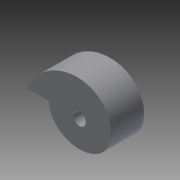
# Autodesk Inventor part: cam 2
Saved by Autodesk Inventor 2014 (Build 180170000, 170)
## iProperties
Created: 2014-05-19
Part Number: cam 2
Material: Generic
Document SubType Name: Modeling
Designer: jyesowitz
Density: 1 g/cm^3
Appearance: Default
Author: jyesowitz
Autodesk Inventor part; units mm, degrees
ref_plane "YZ Plane" through (0, 0, 0) normal (1, 0, 0) x (0, 1, 0)
ref_plane "XZ Plane" through (0, 0, 0) normal (0, 1, 0) x (-1, 0, 0)
ref_plane "XY Plane" through (0, 0, 0) normal (0, 0, 1) x (1, 0, 0)
sketch "Sketch1" plane through (0, 0, 0) normal (0, 0, 1) x (1, 0, 0)
  ellipse E0 centre (-0.0008, -0.0924) end of major axis (23.5196, -0.0924) minor radius 20.2596 (-23.521, 0) -> (22.8214, -4.992) ccw
  line L0 (22.8214, -4.992) -> (30.9811, 23.2074) construction
  line L1 (30.9811, 23.2074) -> (0.0058, 41.0577) construction
  line L2 (0.0058, 41.0577) -> (-30.9314, 23.2159) construction
  line L3 (-30.9314, 23.2159) -> (-40.386, 0) construction
  spline S0 degree 4 poles (22.8214, -4.992) (30.9811, 23.2074) (0.0058, 41.0577) (-30.9314, 23.2159) (-40.386, 0) knots 1 1 1 1 1 2 2 2 2 2
  line L4 (-40.386, 0) -> (-23.521, 0)
  circle A0 centre (-0.0008, -0.0924) radius 4.7625
  point P0 (0, 0)
  dimension "d60" = 23.5204
  dimension "d61" = 20.2596
  dimension "d18" = 40.386
  dimension "d19" = 16.865
  dimension "d29" = 41.0577
  dimension "d30" = 35.7133
  dimension "d31" = 25.0673
  dimension "d32" = 35.7507
  dimension "d33" = 29.3562
  dimension "d43" = 120.074
  dimension "d50" = 9.525
  dimension "d62" = 103.815
  dimension "d63" = 106.138
  constraints: 2 end point, 1 centre point, 1 coincident, 1 horizontal, 8 other
  measures "d18" distance of point (0, 0) L3.end
  measures "d19" distance of L3.end L4.end
  measures "d29" distance of L1.end point (0, 0)
  measures "d30" distance of L1.end L2.end
  measures "d31" distance of L2.end L3.end
  measures "d32" distance of L0.end L1.end
  measures "d33" distance of L0.start L0.end
  measures "d43" angle of L2 L1
  measures "d50" diameter of A0
  measures "d62" angle of L0 L1
  measures "d63" angle of L0 L4
extrude "Extrusion1" add sketch "Sketch1" against normal blind 25.4
body "Solid1"
